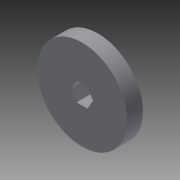
# Autodesk Inventor part: large gear hex
Saved by Autodesk Inventor 2015 (Build 190159000, 159)
## iProperties
Created: 2015-01-17
Part Number: large gear hex
Material: Generic
Document SubType Name: Modeling
Designer: mastkee16
Density: 1 g/cm^3
Appearance: Default
Author: mastkee16
Autodesk Inventor part; units mm, degrees
ref_plane "YZ Plane" through (0, 0, 0) normal (1, 0, 0) x (0, 1, 0)
ref_plane "XZ Plane" through (0, 0, 0) normal (0, 1, 0) x (-1, 0, 0)
ref_plane "XY Plane" through (0, 0, 0) normal (0, 0, 1) x (1, 0, 0)
sketch "Sketch1" plane through (0, 0, 0) normal (0, 0, 1) x (1, 0, 0)
  circle A0 centre (0, 0) radius 29.0893
  dimension "d0" = 58.1787
  constraints: 1 centre point, 1 coincident
  measures "d0" diameter of A0
extrude "Extrusion1" add sketch "Sketch1" along normal blind 10.1905
sketch "Sketch2" plane through (0, 0, 10.1905) normal (0, 0, 1) x (1, 0, 0)
  line L0 (7.0373, 0) -> (3.5186, -6.0945)
  line L1 (3.5186, -6.0945) -> (-3.5186, -6.0945)
  line L2 (-3.5186, -6.0945) -> (-7.0373, 0)
  line L3 (-7.0373, 0) -> (-3.5186, 6.0945)
  line L4 (-3.5186, 6.0945) -> (3.5186, 6.0945)
  line L5 (3.5186, 6.0945) -> (7.0373, 0)
  point P0 (0, 0)
  point P1 (0, 0)
  constraints: 12 end point, 1 coincident, 13 other
extrude "Extrusion2" cut sketch "Sketch2" against normal blind 10.1905
body "Solid1"
